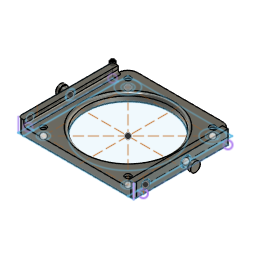
FS80 Bracket v8 (Autodesk Fusion 360 design; units mm, degrees)
Autodesk Fusion 360 part; units mm, degrees
sketch "Schizzo1" plane through (0, 0, 0) normal (0, 0, 1) x (1, 0, 0)
  line L0 (-31.8007, 65.6855) -> (43.3993, 65.6855)
  line L1 (43.3993, 65.6855) -> (43.3993, -9.3145)
  line L2 (43.3993, -9.3145) -> (-31.8007, -9.3145)
  line L3 (-31.8007, -9.3145) -> (-31.8007, 65.6855)
  line L4 (-31.8007, 28.1855) -> (43.3993, 28.1855) construction
  line L5 (5.7993, 65.6855) -> (5.7993, -9.3145) construction
  circle A0 centre (5.7993, 28.1855) radius 30.5
  line L6 (36.2993, -2.3145) -> (-24.7007, -2.3145) construction
  line L7 (-24.7007, -2.3145) -> (-24.7007, 58.6855) construction
  line L8 (-24.7007, 58.6855) -> (36.2993, 58.6855) construction
  line L9 (36.2993, 58.6855) -> (36.2993, -2.3145) construction
  line L10 (36.2993, -2.3145) -> (-24.7007, 58.6855) construction
  line L11 (-24.7007, -2.3145) -> (36.2993, 58.6855) construction
  circle A1 centre (-24.7007, 58.6855) radius 2.1
  circle A2 centre (36.2993, 58.6855) radius 2.1
  circle A3 centre (36.2993, -2.3145) radius 2.1
  circle A4 centre (36.3993, 58.6855) radius 7
  circle A5 centre (-24.7007, -2.3145) radius 2.1
  line L12 (-35.8007, 58.6855) -> (-31.8007, 58.6855)
  line L13 (-31.8007, 58.6855) -> (-31.8007, -2.3145)
  line L14 (-31.8007, -2.3145) -> (-35.8007, -2.3145)
  line L15 (-35.8007, -2.3145) -> (-35.8007, 58.6855)
  line L16 (47.3993, 58.6855) -> (43.3993, 58.6855)
  line L17 (47.3993, -2.3145) -> (47.3993, 58.6855)
  line L18 (43.3993, 58.6855) -> (43.3993, -2.3145)
  line L19 (43.3993, -2.3145) -> (47.3993, -2.3145)
  circle A6 centre (-24.7007, 58.6855) radius 3.6
  circle A7 centre (36.2993, 58.6855) radius 3.6
  circle A8 centre (-24.7007, -2.3145) radius 3.6
  circle A9 centre (36.2993, -2.3145) radius 3.6
  line L20 (-35.8007, -2.3145) -> (-31.8007, -2.3145)
  line L21 (-31.8007, -2.3145) -> (-31.8007, -9.3145)
  line L22 (-31.8007, -9.3145) -> (-35.8007, -9.3145)
  line L23 (-35.8007, -9.3145) -> (-35.8007, -2.3145)
  line L24 (47.3993, -2.3145) -> (43.3993, -2.3145)
  line L25 (43.3993, -2.3145) -> (43.3993, -9.3145)
  line L26 (43.3993, -9.3145) -> (47.3993, -9.3145)
  line L27 (47.3993, -9.3145) -> (47.3993, -2.3145)
  circle A10 centre (-24.8007, 58.6855) radius 7
  point P0 (5.7993, 28.1855)
  point P1 (-24.7007, -2.3145)
  dimension "d1" = 75.2
  dimension "d2" = 75
  dimension "d3" = 61
  dimension "d4" = 61
  dimension "d5" = 61
  dimension "d6" = 4.2
  dimension "d8" = 7
  dimension "d13" = 4
  dimension "d22" = 7.2
  dimension "d60" = 7
  dimension "d70" = 83.2
  constraint horizontal L0
  constraint vertical L1
  constraint horizontal L2
  constraint vertical L3
  constraint midpoint L3 L4.start
  constraint midpoint L1 L4.end
  constraint midpoint L0 L5.start
  constraint midpoint L2 L5.end
  constraint midpoint L4 P0
  constraint horizontal L6
  constraint perpendicular L6 L7
  constraint parallel L6 L8
  constraint parallel L7 L9
  constraint coincident L10 P0
  constraint coincident L11 P0
  constraint coincident P0 A0.centre
  constraint coincident L7.end L8.start
  constraint symmetric L5 A1 A2
  constraint symmetric L4 L7.end P1
  constraint symmetric L4 A2 A3
  constraint tangent L0 A4
  constraint tangent L1 A4
  constraint symmetric L4 A1 A5
  constraint horizontal L12
  constraint vertical L13
  constraint horizontal L14
  constraint vertical L15
  constraint collinear L8 L12
  constraint collinear L3 L13
  constraint collinear L6 L14
  constraint symmetric L5 L12.start L16.start
  constraint symmetric L5 L12.end L16.end
  constraint symmetric L5 L13.end L18.end
  constraint symmetric L5 L14.end L17.start
  constraint concentric A1 A6
  constraint symmetric L5 A6 A7
  constraint symmetric L4 A6 A8
  constraint symmetric L4 A7 A9
  constraint horizontal L20
  constraint vertical L21
  constraint horizontal L22
  constraint vertical L23
  constraint horizontal L24
  constraint vertical L25
  constraint horizontal L26
  constraint vertical L27
  constraint tangent L0 A10
  constraint tangent L3 A10
  measures "d1" distance of L0.start L0.end
  measures "d2" distance of L0.start L2.end
  measures "d3" diameter of A0
  measures "d4" distance of L7.end L8.end
  measures "d5" distance of P1 L7.end
  measures "d6" diameter of A1
  measures "d8" radius of A4
  measures "d13" distance of L13 L15
  measures "d22" diameter of A6
  measures "d60" radius of A10
  measures "d70" distance of L15 L17
extrude "Estrusione1" add sketch "Schizzo1" along normal blind 5.5 contours L0 L1 L2 L3 A4 L13 L18 L21 L25 A10 | A10 | A4 | A6 | A7 | A8 | A9
extrude "Estrusione2" add sketch "Schizzo1" along normal blind 10 contours L3 L12 L13 L14 L15 L20 | L3 L14 L20 L21 L22 L23 | L1 L16 L17 L18 L19 L24 | L1 L19 L24 L25 L26 L27
fillet "Raccordo1" radius 2 1 edges at (43.3993, 24.6855, 5.5)
fillet "Raccordo1" radius 2 1 edges at (-31.8007, 24.6855, 5.5)
extrude "Estrusione3" cut sketch "Schizzo1" along normal blind 4 contours A6 | A7 | A8 | A9
sketch "Schizzo2" plane through (-35.8007, 0, 0) normal (-1, 0, 0) x (0, -1, 0)
  line L0 (-58.6855, 0) -> (9.3145, 0)
  line L1 (9.3145, 10) -> (-58.6855, 10)
  line L2 (-58.6855, 10) -> (-58.6855, 0)
  line L3 (-58.6855, 10) -> (-4.3364, 10) construction
  line L4 (-4.3364, 10) -> (-4.3364, 0) construction
  line L5 (-4.3364, 0) -> (-58.6855, 0) construction
  line L6 (-58.6855, 0) -> (-58.6855, 10) construction
  line L7 (2.3145, 0) -> (-58.6855, 0) construction
  line L8 (-58.6855, 5) -> (-4.3364, 5) construction
  circle A0 centre (-28.1855, 5) radius 2.9
  circle A1 centre (-28.1855, 5) radius 3.5
  line L9 (9.3145, 0) -> (9.3145, 10)
  circle A2 centre (0.8145, 5) radius 2.9
  dimension "d25" = 10
  dimension "d27" = 5.8
  dimension "d28" = 7
  dimension "d56" = 5.8
  dimension "d64" = 30.5
  dimension "d65" = 29
  constraint horizontal L3
  constraint vertical L4
  constraint horizontal L5
  constraint vertical L6
  constraint coincident L1.end L2.start
  constraint collinear L5 L7
  constraint midpoint L6 L8.start
  constraint midpoint L4 L8.end
  constraint coincident L8 A2.centre
  constraint coincident A0.centre A1.centre
  measures "d25" distance of L3 L7
  measures "d27" diameter of A0
  measures "d28" diameter of A1
  measures "d56" diameter of A2
  measures "d64" distance of L6 A0.centre
  measures "d65" distance of A0.centre A2.centre
extrude "Estrusione4" add sketch "Schizzo2" along normal blind 7 contours A0
extrude "Estrusione5" add sketch "Schizzo2" against normal blind 2 from surface at 7 contours A1
fillet "Raccordo4" radius 0.5 1 edges at (-35.8007, 30.8893, 6.0487)
extrude "Estrusione10" cut sketch "Schizzo2" against normal blind 3.5 contours A2
sketch "Schizzo3" plane through (47.3993, 0, 0) normal (1, 0, 0) x (0, 1, 0)
  line L0 (-9.3145, 0) -> (58.6855, 0)
  line L1 (58.6855, 0) -> (58.6855, 10)
  line L2 (58.6855, 10) -> (-9.3145, 10)
  line L3 (-2.3145, 10) -> (58.6855, 10) construction
  line L4 (58.6855, 10) -> (58.6855, 0) construction
  line L5 (58.6855, 0) -> (-2.3145, 0) construction
  line L6 (-2.3145, 0) -> (-2.3145, 10) construction
  line L7 (-2.3145, 0) -> (58.6855, 0) construction
  line L8 (-2.3145, 5) -> (58.6855, 5) construction
  circle A0 centre (28.1855, 5) radius 2.9
  circle A1 centre (28.1855, 5) radius 3.5
  line L9 (-9.3145, 10) -> (-9.3145, 0)
  circle A2 centre (-0.8145, 5) radius 2.9
  dimension "d36" = 5.8
  dimension "d37" = 7
  dimension "d49" = 5.8
  dimension "d50" = 29
  dimension "d51" = 30.5
  constraint horizontal L3
  constraint vertical L4
  constraint horizontal L5
  constraint vertical L6
  constraint collinear L5 L7
  constraint collinear L2 L3
  constraint collinear L1 L4
  constraint midpoint L6 L8.start
  constraint midpoint L4 L8.end
  constraint concentric A0 A1
  constraint coincident L8 A2.centre
  measures "d36" diameter of A0
  measures "d37" diameter of A1
  measures "d49" diameter of A2
  measures "d50" distance of A0.centre A2.centre
  measures "d51" distance of L4 A0.centre
extrude "Estrusione6" add sketch "Schizzo3" along normal blind 7 contours A0
extrude "Estrusione7" add sketch "Schizzo3" against normal blind 2 from surface at 7 contours A1
fillet "Raccordo5" radius 0.5 1 edges at (47.3993, 25.4818, 6.0487)
extrude "Estrusione11" cut sketch "Schizzo3" against normal blind 3.5 contours A2
fillet "Raccordo6" radius 2 1 edges at (-35.8007, -9.3145, 5)
fillet "Raccordo6" radius 2 1 edges at (47.3993, -9.3145, 5)
fillet "Raccordo7" radius 2 1 edges at (-22.6367, 39.2148, 5.5)
equation "d1 = 75 mm + 0.2 mm"
equation "d51 = ( 61 / 2 ) * 1 mm"
equation "d64 = ( 61 / 2 ) * 1 mm"
